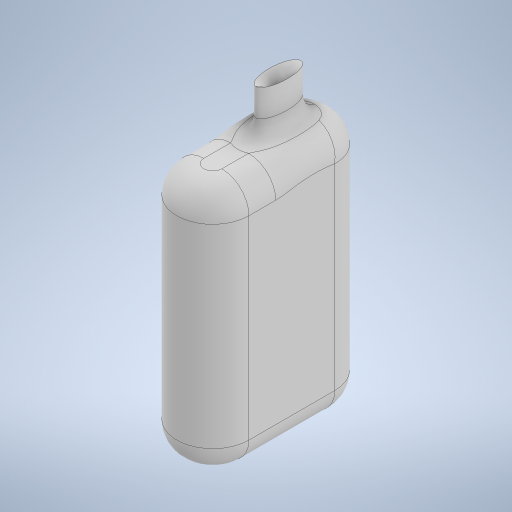
# Autodesk Inventor part: PUFIK_1
Saved by Autodesk Inventor 2023 (Build 270158000, 158)
## iProperties
Created: 2024-04-21
Part Number: PUFIK_1
Material: Generic
Document SubType Name: Modeling
Designer: VRACOVSKÝ
Density: 1 g/cm^3
Appearance: Default
Author: vraco
Autodesk Inventor part; units mm, degrees
ref_plane "YZ Plane" through (0, 0, 0) normal (1, 0, 0) x (0, 1, 0)
ref_plane "XZ Plane" through (0, 0, 0) normal (0, 1, 0) x (-1, 0, 0)
ref_plane "XY Plane" through (0, 0, 0) normal (0, 0, 1) x (1, 0, 0)
sketch "Sketch1" plane through (0, 0, 0) normal (0, 1, 0) x (-1, 0, 0)
  line L0 (0, -24.5) -> (0, 24.5) projected
  line L1 (-11.2, 0) -> (11.2, 0) projected
  line L2 (0, 17.5) -> (0, -17.5) construction
  line L3 (-8, 9.5) -> (-8, -9.5)
  line L4 (8, -9.5) -> (8, 9.5)
  arc A0 (8, 9.5) -> (-8, 9.5) centre (0, 9.5) ccw
  arc A1 (-8, -9.5) -> (8, -9.5) centre (0, -9.5) ccw
  point P0 (0, 0)
  point P1 (0, 0)
  dimension "d0" = 35
  dimension "d1" = 16
  constraints: 8 end point, 8 point on circle, 4 point on line, 4 tangent, 2 centre point, 1 midpoint, 1 parallel, 1 symmetric about line
  measures "d0" distance of point (0, -17.5) point (0, 17.5)
  measures "d1" distance between parallel lines of L3 L4
extrude "Extrusion1" add sketch "Sketch1" along normal blind 55
sketch "Sketch2" plane through (0, 55, 0) normal (0, 1, 0) x (1, 0, 0)
  line L0 (0, 24.5) -> (0, -24.5) projected
  line L1 (11.2, 0) -> (-11.2, 0) projected
  ellipse E0 centre (0, 5) end of major axis (0, 10) minor radius 2
  point P0 (0, 0)
  dimension "d4" = 2
  dimension "d5" = 5
  constraints: 1 point on line, 1 vertical alignment, 2 other
extrude "Extrusion2" add sketch "Sketch2" along normal blind 10
fillet "Fillet1" radius 4 1 edges at (0, 55, 0)
fillet "Fillet2" radius 6 3 edges at (8, 55, 0) (-8, 55, 0) (0, 55, 17.5)
fillet "Fillet3" radius 6 4 edges at (0, 0, -17.5) (-8, 0, 0) (0, 0, 17.5) (8, 0, 0)
sketch "Sketch3" plane through (0, 65, 0) normal (0, 1, 0) x (1, 0, 0)
  ellipse E0 centre (0, 5) end of major axis (0, 10) minor radius 2 projected
  point P0 (0, 0)
  constraints: 1 coincident, 1 vertical alignment
hole "Hole1" at (0, 65, -5) direction (0, -1, 0) diameter 2 depth 8 tip angle 118
fillet "Fillet4" radius 6 1 edges at (0, 65, -6)
body "Solid1"
